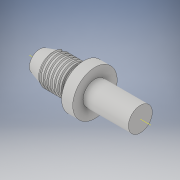
# Autodesk Inventor part: Table Leg
Saved by Autodesk Inventor 2018 (Build 220112000, 112)
## iProperties
Created: 2019-03-13
Part Number: Table Leg
Material: Generic
Document SubType Name: Modeling
Designer: 10036316
Density: 1 g/cm^3
Appearance: Default
Author: 10036316
## iProperties of the stored document Table Leg_3DPrint.ipt
Created: 2019-03-14
Part Number: Table Leg_3DPrint
Material: Generic
Document SubType Name: Modeling
Designer: 10036316
Density: 1 g/cm^3
Appearance: Default
Author: 10036316
Autodesk Inventor part; units mm, degrees
ref_plane "YZ Plane" through (0, 0, 0) normal (1, 0, 0) x (0, 1, 0)
sketch "Sketch3" plane through (0, 0, 0) normal (0, 0, 1) x (1, 0, 0)
  circle A0 centre (0, 0) radius 12.4219
  dimension "d4" = 24.8437
  constraints: 1 centre point, 1 coincident
  measures "d4" diameter of A0
extrude "Extrusion2" add sketch "Sketch3" along normal blind 6.2535
sketch "Sketch4" plane through (0, 0, 0) normal (0, 0, -1) x (-1, 0, 0)
  circle A0 centre (0, 0) radius 6.698
  dimension "d7" = 13.396
  constraints: 1 centre point, 1 coincident
  measures "d7" diameter of A0
extrude "Extrusion3" add sketch "Sketch4" along normal blind 25.4
sketch "Sketch5" plane through (0, 0, 6.2535) normal (0, 0, 1) x (1, 0, 0)
  circle A0 centre (0, 0) radius 7.9477
  dimension "d10" = 15.8953
  constraints: 1 centre point, 1 coincident
  measures "d10" diameter of A0
extrude "Extrusion4" add sketch "Sketch5" along normal blind 17.3253
ref_plane "Work Plane1" through (0, 0, 30.9423) normal (0, 0, 1) x (1, 0, 0)
sketch "Sketch7" plane through (0, 0, 30.9423) normal (0, 0, 1) x (1, 0, 0)
  circle A0 centre (0, 0) radius 5.7238
  constraints: 1 centre point, 1 coincident
loft "Loft1" add profiles "Sketch7" section 1 edges at (-7.9477, 0, 23.5788)
sketch "Sketch9" plane through (0, 0, 6.2535) normal (0, 0, 1) x (1, 0, 0)
  point P0 (0, 0)
  point P1 (0, -7.9375)
sketch3d "3D Sketch3"
sketch3d "3D Sketch4"
ref_plane "Work Plane5" through (0.4877, -7.9375, 11.9267) normal (1, 0, 0) x (0, 1, 0)
sketch "Sketch14" plane through (0.4877, -7.9375, 11.9267) normal (1, 0, 0) x (0, 1, 0)
  line L0 (-0.0102, -5.6732) -> (15.8852, -5.6732) projected
  line L1 (15.8852, -5.6732) -> (15.8852, -4.9793)
  line L2 (15.8852, -4.9793) -> (14.8304, -5.4704)
  line L3 (14.8304, -5.4704) -> (15.8852, -5.6732)
  line L4 (15.8852, -4.9793) -> (16.4561, -5.2249)
  line L5 (16.4561, -5.2249) -> (15.8852, -5.6732)
  point P0 (7.9375, -11.9267)
  constraints: 10 end point, 1 vertical
coil "Coil1" sketch "Sketch14" operation add axis through (0, 0, 6.2535) along (0, 0, 1) pitch 2.032 turns 8.1 hand right contours L1 L4 L5
body "Solid2"
